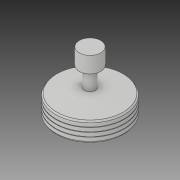
# Autodesk Inventor part: Top1
Saved by Autodesk Inventor 2018 (Build 220112000, 112)
## iProperties
Created: 2017-12-12
Part Number: Top1
Material: Generic
Document SubType Name: Modeling
Designer: Rus
Density: 1 g/cm^3
Appearance: Default
Author: Rus
Autodesk Inventor part; units mm, degrees
ref_plane "YZ Plane" through (0, 0, 0) normal (1, 0, 0) x (0, 1, 0)
ref_plane "XZ Plane" through (0, 0, 0) normal (0, 1, 0) x (-1, 0, 0)
ref_plane "XY Plane" through (0, 0, 0) normal (0, 0, 1) x (1, 0, 0)
sketch "Sketch1" plane through (0, 0, 0) normal (0, 0, 1) x (1, 0, 0)
  line L0 (0, 0) -> (0, 28.575)
  line L1 (0, 0) -> (0, -6.35)
  line L2 (0, 28.575) -> (0, 38.1)
  line L3 (6.35, 28.575) -> (6.35, 38.1)
  line L4 (6.35, 38.1) -> (0, 38.1)
  line L5 (3.175, 17.0324) -> (0, 17.0324) construction
  line L6 (6.35, 28.575) -> (3.175, 28.575)
  line L7 (3.175, 28.575) -> (0, 28.575) construction
  line L8 (0, 0) -> (3.175, 0) construction
  line L9 (3.175, 0) -> (17.91, 0) construction
  line L10 (19.6531, 2.9055) -> (20.32, 3.858)
  line L11 (0, -6.35) -> (3.175, -4.2333)
  line L12 (3.175, -4.2333) -> (3.175, 0)
  line L13 (3.175, 0) -> (19.6531, 2.9055)
  line L14 (3.175, 28.575) -> (3.175, 17.2411)
  line L15 (20.32, 13.383) -> (19.6531, 14.3355)
  line L16 (19.6531, 14.3355) -> (3.175, 17.2411)
  line L17 (20.32, 8.7793) -> (20.1613, 8.6205) construction
  line L18 (20.1613, 8.6205) -> (20.32, 8.4618) construction
  arc A0 (6.35, 38.1) -> (0, 40.0262) centre (0, 28.5962) ccw
  line L19 (20.32, 6.3187) -> (20.1612, 6.1599) construction
  line L20 (20.1612, 6.1599) -> (20.32, 6.0012) construction
  line L21 (20.32, 10.9224) -> (20.1612, 11.0812) construction
  line L22 (20.1612, 11.0812) -> (20.32, 11.2399) construction
  line L23 (20.32, 3.858) -> (20.32, 6.0012)
  line L24 (20.32, 6.3187) -> (20.32, 8.4618)
  line L25 (20.32, 8.7793) -> (20.32, 10.9224)
  line L26 (20.32, 11.2399) -> (20.32, 13.383)
  line L27 (20.32, 6.0012) -> (20.32, 6.3187) construction
  line L28 (20.32, 8.4618) -> (20.32, 8.7793) construction
  line L29 (20.32, 10.9224) -> (20.32, 11.2399) construction
  arc A1 (20.32, 11.2399) -> (20.32, 10.9224) centre (20.4787, 11.0812) ccw
  arc A2 (20.32, 8.7793) -> (20.32, 8.4618) centre (20.4787, 8.6205) ccw
  arc A3 (20.32, 6.3187) -> (20.32, 6.0012) centre (20.4787, 6.1599) ccw
  dimension "d5" = 44.45
  dimension "d6" = 9.525
  dimension "d7" = 6.35
  dimension "d12" = 2.1167
  dimension "d13" = 3.175
  dimension "d15" = 4.2333
  dimension "d24" = 10
  dimension "d28" = 3.175
  dimension "d31" = 110
  dimension "d32" = 100
  dimension "d35" = 11.43
  dimension "d36" = 0.3175
  dimension "d37" = 9.525
  dimension "d40" = 11.43
  dimension "d42" = 20.32
  constraints: 61 end point, 11 vertical, 9 equal length, 8 point on circle, 4 centre point, 4 perpendicular, 3 collinear, 3 horizontal, 3 point on line, 2 equal radius, 1 line through centre, 1 parallel, 1 tangent, 1 vertical alignment
  measures "d5" distance of L2.end L1.end
  measures "d6" distance of L3.start L3.end
  measures "d7" distance between parallel lines of L2 L3
  measures "d12" vertical distance of L11.end L1.end
  measures "d13" horizontal distance of L1.end L11.end
  measures "d15" distance from line of L9 L11.end
  measures "d24" angle of L13 L9
  measures "d28" distance of L3.start L6.end
  measures "d31" angle of L15 L10
  measures "d32" angle of L14 L16
  measures "d35" distance of L15.end L10.start
  measures "d36" distance of L17.start L18.end
  measures "d37" distance of L15.start L10.end
  measures "d40" radius of A0
  measures "d42" distance between parallel lines of L24 L0
revolve "Revolution1" add sketch "Sketch1" angle 360 about axis through (0, 28.575, 0) along (0, -1, 0)
body "Solid1"
